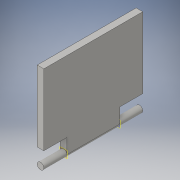
# Autodesk Inventor part: gpsDoor
Saved by Autodesk Inventor 2016 (Build 200138000, 138)
## iProperties
Created: 2016-10-13
Part Number: gpsDoor
Material: Generic
Document SubType Name: Modeling
Designer: lachesis
Density: 1 g/cm^3
Appearance: Default
Author: lachesis
Autodesk Inventor part; units mm, degrees
ref_plane "YZ Plane" through (0, 0, 0) normal (1, 0, 0) x (0, 1, 0)
ref_plane "XZ Plane" through (0, 0, 0) normal (0, 1, 0) x (-1, 0, 0)
ref_plane "XY Plane" through (0, 0, 0) normal (0, 0, 1) x (1, 0, 0)
sketch "Sketch1" plane through (0, 0, 0) normal (0, 0, 1) x (1, 0, 0)
  circle A0 centre (0, 0) radius 1
  dimension "d0" = 2
  constraints: 1 centre point, 1 coincident
  measures "d0" diameter of A0
extrude "Extrusion1" add sketch "Sketch1" along normal blind 30
ref_plane "Work Plane1" through (0, 0, 23) normal (0, 0, 1) x (1, 0, 0)
ref_plane "Work Plane2" through (0, 0, 7) normal (0, 0, -1) x (-1, 0, 0)
sketch "Sketch2" plane through (0, 0, 23) normal (0, 0, 1) x (1, 0, 0)
  circle A0 centre (0, 0) radius 1 projected
  line L0 (1, 0) -> (-1, 0)
  line L1 (-1, 0) -> (-1, 26)
  line L2 (-1, 26) -> (1, 26)
  line L3 (1, 26) -> (1, 0)
  dimension "d7" = 26
  constraints: 8 end point, 2 parallel, 2 point on circle, 1 coincident, 1 horizontal, 1 midpoint, 1 perpendicular
  measures "d7" distance from line of point (0, 0) L2
extrude "Extrusion2" add sketch "Sketch2" against normal up to surface (16 mm away) contours A0 L1 L2 L3
sketch "Sketch3" plane through (1, 0, 23) normal (1, 0, 0) x (0, 0, -1)
  line L0 (16, 0) -> (16, 26) projected
  line L1 (0, 26) -> (16, 26) projected
  line L2 (0, 0) -> (0, 26) projected
  line L3 (16, 0) -> (0, 0) projected
  line L4 (0, 26) -> (-7, 26)
  line L5 (-7, 26) -> (-7, 4.5)
  line L6 (-7, 4.5) -> (0, 4.5)
  line L7 (0, 4.5) -> (0, 26)
  line L8 (16, 0) -> (16, 26) projected
  line L9 (16, 26) -> (23, 26)
  line L10 (23, 26) -> (23, 4.5)
  line L11 (23, 4.5) -> (16, 4.5)
  line L12 (16, 4.5) -> (16, 26)
  line L13 (23, -1) -> (23, 1) projected
  line L14 (-7, 1) -> (-7, -1) projected
  line L15 (16, 0) -> (0, 0) projected
  line L16 (16, 0) -> (16, 0) projected
  line L17 (16, 0) -> (0, 0) projected
  line L18 (0, 0) -> (0, 0) projected
  point P0 (23, 0)
  point P1 (19.5, 4.5)
  point P2 (-3.5, 4.5)
  point P3 (23, 0)
  point P4 (23, 15.25)
  point P5 (-7, 15.25)
  point P6 (-7, 0)
  dimension "d10" = 3.5
  constraints: 16 end point, 6 midpoint, 4 parallel, 2 horizontal, 2 perpendicular, 2 vertical alignment, 1 horizontal alignment
  measures "d10" distance from line of L13.end L11
extrude "Extrusion3" add sketch "Sketch3" against normal up to surface (2 mm away) contours L0 L9 L10 L11 | L6 L5 L4 L2
body "Solid1"
